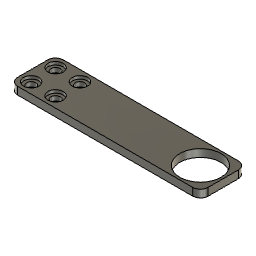
_Motorised arm support bracket.2e501b18-44f0-4462-bb6e-af1a0b4020e3 (Autodesk Fusion 360 design; units mm, degrees)
Autodesk Fusion 360 part; units mm, degrees
sketch "Sketch1" plane through (0, 0, 0) normal (0, 0, 1) x (1, 0, 0)
  line L0 (0, 0) -> (125, 0)
  line L1 (125, 0) -> (125, 30)
  line L2 (125, 30) -> (0, 30)
  line L3 (0, 30) -> (0, 0)
  dimension "d1" = 125
  dimension "d2" = 30
  constraint horizontal L0
  constraint vertical L1
  constraint horizontal L2
  constraint vertical L3
  constraint coincident L0.start L3.end
  measures "d1" distance of L0.start L0.end
  measures "d2" distance of L0.start L2.end
extrude "Extrude1" add sketch "Sketch1" along normal blind 5
sketch "Sketch2" plane through (0, 0, 5) normal (0, 0, 1) x (-1, 0, 0)
  line L0 (0, -30) -> (0, 0)
  line L1 (0, 0) -> (-125, 0)
  line L2 (-125, 0) -> (-125, -30)
  line L3 (-125, -30) -> (0, -30)
  circle A0 centre (-110, -15) radius 13.5
  dimension "d5" = 27
  measures "d5" diameter of A0
extrude "Extrude2" cut sketch "Sketch2" against normal blind 5 contours A0
sketch "Sketch3" plane through (0, 0, 5) normal (0, 0, 1) x (-1, 0, 0)
  circle A0 centre (-110, -15) radius 13.5
  line L0 (0, -30) -> (0, 0)
  line L1 (0, 0) -> (-125, 0)
  line L2 (-125, 0) -> (-125, -30)
  line L3 (-125, -30) -> (0, -30)
  circle A1 centre (-7, -23) radius 3
  circle A2 centre (-7, -7) radius 3
  circle A3 centre (-23, -23) radius 3
  circle A4 centre (-23, -7) radius 3
  dimension "d8" = 6
  dimension "d9" = 6
  dimension "d10" = 6
  dimension "d11" = 6
  measures "d8" diameter of A1
  measures "d9" diameter of A2
  measures "d10" diameter of A3
  measures "d11" diameter of A4
extrude "Extrude3" cut sketch "Sketch3" against normal blind 5 contours A1 | A2 | A3 | A4
sketch "Sketch4" plane through (0, 0, 5) normal (0, 0, 1) x (-1, 0, 0)
  circle A0 centre (-23, -7) radius 3
  circle A1 centre (-23, -23) radius 3
  circle A2 centre (-7, -7) radius 3
  circle A3 centre (-7, -23) radius 3
  circle A4 centre (-110, -15) radius 13.5
  line L0 (0, -30) -> (0, 0)
  line L1 (0, 0) -> (-125, 0)
  line L2 (-125, 0) -> (-125, -30)
  line L3 (-125, -30) -> (0, -30)
  circle A5 centre (-7, -23) radius 5
  circle A6 centre (-23, -23) radius 5
  circle A7 centre (-7, -7) radius 5
  circle A8 centre (-23, -7) radius 5
  dimension "d14" = 10
  dimension "d15" = 10
  dimension "d16" = 10
  dimension "d17" = 10
  constraint concentric A3 A5
  constraint concentric A1 A6
  constraint concentric A2 A7
  constraint concentric A0 A8
  measures "d14" diameter of A5
  measures "d15" diameter of A6
  measures "d16" diameter of A7
  measures "d17" diameter of A8
extrude "Extrude4" cut sketch "Sketch4" against normal blind 2 contours A5 | A6 | A7 | A8
fillet "Fillet1" radius 5 4 edges at (125, 30, 2.5) (125, 0, 2.5) (0, 0, 2.5) (0, 30, 2.5)
